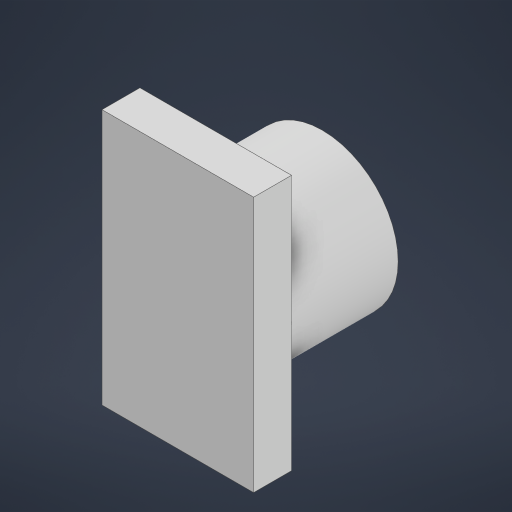
# Autodesk Inventor part: ButtonInsert
Saved by Autodesk Inventor 2023 (Build 270158000, 158)
## iProperties
Created: 2023-01-26
Part Number: ButtonInsert
Material: Generic
Document SubType Name: Modeling
Designer: jevan
Density: 1 g/cm^3
Appearance: Default
Author: jevan
Autodesk Inventor part; units mm, degrees
ref_plane "YZ Plane" through (0, 0, 0) normal (1, 0, 0) x (0, 1, 0)
ref_plane "XZ Plane" through (0, 0, 0) normal (0, 1, 0) x (-1, 0, 0)
ref_plane "XY Plane" through (0, 0, 0) normal (0, 0, 1) x (1, 0, 0)
sketch "Sketch1" plane through (0, 0, 0) normal (0, 0, 1) x (1, 0, 0)
  line L0 (0, 0) -> (-3.2, 0)
  line L1 (-3.2, 0) -> (-3.2, 5.4)
  line L2 (-3.2, 5.4) -> (0, 5.4)
  line L3 (0, 5.4) -> (0, 0)
  circle A0 centre (-1.6, 2.7) radius 1.2
  line L4 (0, 2.7) -> (-1.6, 2.7)
  circle A1 centre (-1.6, 2.7) radius 1.6
  line L5 (-1.6, 2.7) -> (-3.2, 2.7)
  point P0 (-2.2, 1.7802)
  point P1 (0, 2.7)
  point P2 (0, 1.7802)
  dimension "d0" = 3.2
  dimension "d1" = 5.4
  dimension "d9" = 3.2
  dimension "d10" = 0.4
  constraints: 12 end point, 3 horizontal, 2 centre point, 2 midpoint, 2 parallel, 1 coincident, 1 collinear, 1 perpendicular
  measures "d0" distance of L1.end L2.end
  measures "d1" distance of L0.end L1.end
  measures "d9" diameter of A1
  measures "d10" radial gap between concentric circles of A1 A0
extrude "Extrusion1" add sketch "Sketch1" along normal blind 0.8
extrude "Extrusion2" add sketch "Sketch1" against normal blind 2.5 contours A1 L5 A0 L4 | L4 A0 L5 A1 | L4 L5 A0 | A0 L5 L4
chamfer "Chamfer1" distance 0.8 distance2 0.25 1 edges at (-3.2, 2.7, -2.5) measured on face at (-1.6496, 3.1082, -2.5)
body "Solid1"
